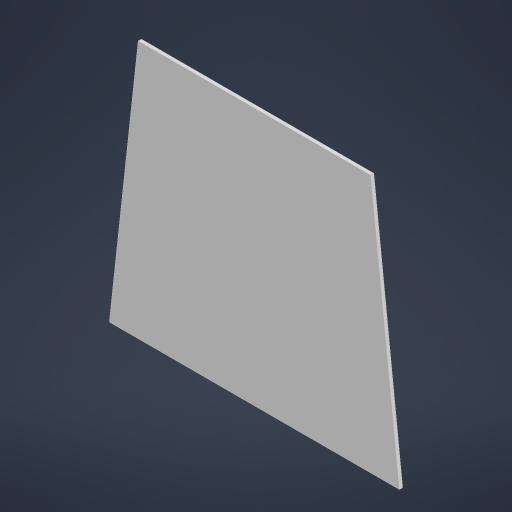
# Autodesk Inventor part: Langbektang houder
Saved by Autodesk Inventor 2023.2 (Build 272271000, 271)
## iProperties
Created: 2020-09-09
Part Number: Langbektang houder
Material: Generic
Document SubType Name: Modeling
Designer: nathan.bollaert
Density: 1 g/cm^3
Appearance: Clear
Author: nathan.bollaert
Autodesk Inventor part; units mm, degrees
ref_plane "YZ Plane" through (0, 0, 0) normal (1, 0, 0) x (0, 1, 0)
ref_plane "XZ Plane" through (0, 0, 0) normal (0, 1, 0) x (-1, 0, 0)
ref_plane "XY Plane" through (0, 0, 0) normal (0, 0, 1) x (1, 0, 0)
sketch "Sketch1" plane through (0, 0, 0) normal (0, 0, 1) x (1, 0, 0)
  line L0 (0, 0) -> (14, 125.1947)
  line L1 (14, 125.1947) -> (104, 125.1947)
  line L2 (104, 125.1947) -> (118, 0)
  line L3 (16, 0) -> (28, 0)
  line L4 (28, 0) -> (28, -4)
  line L5 (28, -4) -> (16, -4)
  line L6 (16, -4) -> (16, 0)
  line L7 (66, 0) -> (78, 0)
  line L8 (78, 0) -> (78, -4)
  line L9 (78, -4) -> (66, -4)
  line L10 (66, -4) -> (66, 0)
  line L11 (40, 0) -> (52, 0)
  line L12 (52, 0) -> (52, -4)
  line L13 (52, -4) -> (40, -4)
  line L14 (40, -4) -> (40, 0)
  line L15 (90, 0) -> (102, 0)
  line L16 (102, 0) -> (102, -4)
  line L17 (102, -4) -> (90, -4)
  line L18 (90, -4) -> (90, 0)
  line L19 (78, 0) -> (90, 0)
  line L20 (28, 0) -> (40, 0)
  line L21 (102, 0) -> (118, 0)
  line L22 (16, 0) -> (0, 0)
  line L23 (52, 0) -> (66, 0)
  line L24 (102, -4) -> (118.4473, -4)
  line L25 (118.4473, -4) -> (118, 0)
  dimension "d229" = 90
  dimension "d232" = 16
  dimension "d233" = 12
  dimension "d234" = 12
  dimension "d235" = 4
  dimension "d239" = 14
  dimension "d241" = 130
  constraints: 52 end point, 9 equal length, 9 horizontal, 8 parallel, 4 perpendicular, 3 collinear
  measures "d229" distance of L0.end L1.end
  measures "d232" horizontal distance of L0.start L5.end
  measures "d233" distance of L4.end L5.end
  measures "d234" distance of L3.end L11.start
  measures "d235" distance of L5.end L3.start
  measures "d239" distance between parallel lines of L10 L12
  measures "d241" distance of L24.end L1.end
extrude "Extrusion1" add sketch "Sketch1" against normal blind 4 contours L0 L1 L2 L21 L15 L19 L7 L23 L11 L20 L3 L22 | L3 L4 L5 L6 | L11 L12 L13 L14 | L16 L17 L18 L15 | L7 L8 L9 L10
sketch "Sketch2" plane through (0, 0, 0) normal (0, 0, 1) x (1, 0, 0)
  line L0 (9, 25) -> (109, 25)
  line L1 (109, 25) -> (109, 8)
  line L2 (109, 8) -> (9, 8)
  line L3 (9, 8) -> (9, 25)
  line L4 (22.9441, 115.1947) -> (95.0559, 115.1947)
  line L5 (95.0559, 115.1947) -> (104.002, 35.1947)
  line L6 (104.002, 35.1947) -> (13.998, 35.1947)
  line L7 (13.998, 35.1947) -> (22.9441, 115.1947)
  line L8 (118, 0) -> (104, 125.1947) projected
  line L9 (14, 125.1947) -> (0, 0) projected
  line L10 (104, 125.1947) -> (14, 125.1947) projected
  line L11 (59, 125.1947) -> (59, 0)
  line L12 (52, 0) -> (66, 0) projected
  dimension "d242" = 100
  dimension "d243" = 17
  dimension "d245" = 8
  dimension "d246" = 10
  dimension "d247" = 80
  dimension "d249" = 10
  constraints: 18 end point, 5 parallel, 2 horizontal, 2 midpoint, 1 perpendicular, 2 other
  measures "d242" distance of L1.end L2.end
  measures "d243" distance of L0.end L1.end
  measures "d245" vertical distance of L9.end L1.end
  measures "d246" distance between parallel lines of L10 L4
  measures "d247" distance between parallel lines of L4 L6
  measures "d249" distance between parallel lines of L9 L7
extrude "Extrusion2" cut sketch "Sketch2" against normal blind 4
extrude "Extrusion3" add sketch "Sketch2" against normal blind 2.5 contours L4 L11 L6 L7 | L4 L5 L6 L11
extrude "Extrusion4" cut sketch "Sketch2" against normal blind 1.5 contours L4 L11 L6 L7 | L4 L5 L6 L11
extrude "Extrusion5" cut sketch "Sketch2" against normal blind 2.5 contours L4 L11 L6 L7 | L4 L5 L6 L11 keep common part
body "Solid5"
